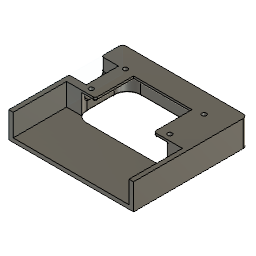
co2_fascia (Autodesk Fusion 360 design; units mm, degrees)
part number: 2026-03-11-11-56-11-354
Autodesk Fusion 360 part; units mm, degrees
note: some values were not read from the file. Chosen so that the rebuilt part matches the saved one: which face or edge a step refers to. Set by a fixed rule: which sketch regions a step uses.
sketch "Sketch1" plane through (0, 0, 0) normal (0, 0, 1) x (1, 0, 0)
  line L0 (0, 0) -> (62, 0)
  line L1 (62, 0) -> (62, 56.5)
  line L2 (62, 56.5) -> (0, 56.5)
  line L3 (0, 56.5) -> (0, 0)
  dimension "d1" = 62
  dimension "d2" = 56.5
  constraint horizontal L0
  constraint vertical L1
  constraint horizontal L2
  constraint vertical L3
  constraint coincident L0.start L3.end
  measures "d1" distance of L0.start L0.end
  measures "d2" distance of L0.start L2.end
extrude "Extrude1" add sketch "Sketch1" along normal blind 13
sketch "Sketch2" plane through (0, 0, 13) normal (0, 0, 1) x (-1, 0, 0)
  line L0 (0, -56.5) -> (0, 0)
  line L1 (0, 0) -> (-62, 0)
  line L2 (-62, 0) -> (-62, -56.5)
  line L3 (-62, -56.5) -> (0, -56.5)
  line L4 (-2.25, -26.5) -> (-59.75, -26.5)
  line L5 (-59.75, -26.5) -> (-59.75, 0.5)
  line L6 (-59.75, 0.5) -> (-2.25, 0.5)
  line L7 (-2.25, 0.5) -> (-2.25, -26.5)
  dimension "d5" = 57.5
  dimension "d6" = 27
  dimension "d7" = 30
  dimension "d8" = 2.25
  constraint horizontal L4
  constraint vertical L5
  constraint horizontal L6
  constraint vertical L7
  measures "d5" distance of L4.start L4.end
  measures "d6" distance of L4.start L6.end
  measures "d7" distance of L3 L4
  measures "d8" distance of L0 L7
extrude "Extrude2" cut sketch "Sketch2" against normal blind 11 contours L1 L4 L5 L7 | L1 L5 L6 L7
sketch "Sketch3" plane through (0, 0, 13) normal (0, 0, 1) x (-1, 0, 0)
  line L0 (-59.75, -26.5) -> (-59.75, 0)
  line L1 (-59.75, 0) -> (-62, 0)
  line L2 (-62, 0) -> (-62, -56.5)
  line L3 (-62, -56.5) -> (0, -56.5)
  line L4 (0, -56.5) -> (0, 0)
  line L5 (0, 0) -> (-2.25, 0)
  line L6 (-2.25, 0) -> (-2.25, -26.5)
  line L7 (-2.25, -26.5) -> (-59.75, -26.5)
  point P0 (-11.5, -46.5)
  point P1 (-50.5, -46.5)
  point P2 (-11.5, -29.5)
  point P3 (-50.5, -29.5)
  dimension "d11" = 10
  dimension "d12" = 11.5
  dimension "d15" = -39
  dimension "d16" = 17
  measures "d11" distance of L3 P0
  measures "d12" distance of L4 P0
hole "Hole1" at (50.5, 46.5, 13) at (50.5, 29.5, 13) at (11.5, 29.5, 13) at (11.5, 46.5, 13) direction (0, 0, -1) diameter 2.2 end through all
sketch "Sketch4" plane through (0, 0, 0) normal (0, 0, -1) x (1, 0, 0)
  circle A0 centre (11.5, -29.5) radius 1.1
  circle A1 centre (50.5, -46.5) radius 1.1
  circle A2 centre (50.5, -29.5) radius 1.1
  circle A3 centre (11.5, -46.5) radius 1.1
  line L0 (0, 0) -> (0, -56.5)
  line L1 (0, -56.5) -> (62, -56.5)
  line L2 (62, -56.5) -> (62, 0)
  line L3 (62, 0) -> (0, 0)
  line L4 (47.75, -51.275) -> (14.2, -51.275)
  line L5 (7.7, -44.775) -> (7.7, -31.225)
  line L6 (14.2, -24.725) -> (47.75, -24.725)
  line L7 (54.25, -31.225) -> (54.25, -44.775)
  arc A4 (47.75, -51.275) -> (54.25, -44.775) centre (47.75, -44.775) ccw
  arc A5 (7.7, -44.775) -> (14.2, -51.275) centre (14.2, -44.775) ccw
  arc A6 (14.2, -24.725) -> (7.7, -31.225) centre (14.2, -31.225) ccw
  arc A7 (54.25, -31.225) -> (47.75, -24.725) centre (47.75, -31.225) ccw
  point P0 (54.25, -51.275)
  point P1 (7.7, -51.275)
  point P2 (54.25, -24.725)
  dimension "d19" = 46.55
  dimension "d20" = 26.55
  dimension "d21" = 7.75
  dimension "d22" = 4.775
  dimension "d35" = 6.5
  constraint horizontal L4
  constraint vertical L5
  constraint horizontal L6
  constraint vertical L7
  constraint coincident P0 L7
  constraint coincident P0 L4
  constraint tangent L7 A4
  constraint tangent L4 A4
  constraint coincident P1 L4
  constraint coincident P1 L5
  constraint tangent L4 A5
  constraint tangent L5 A5
  constraint equal A4 A5
  constraint tangent L5 A6
  constraint tangent L6 A6
  constraint equal A4 A6
  constraint coincident P2 L6
  constraint coincident P2 L7
  constraint tangent L6 A7
  constraint tangent L7 A7
  constraint equal A4 A7
  measures "d19" distance of P0 P1
  measures "d20" distance of P0 P2
  measures "d21" distance of L2 L7
  measures "d22" distance of A1.centre L4
  measures "d35" radius of A4
extrude "Extrude3" cut sketch "Sketch4" against normal blind 11 contours L4 L5 L6 L7 A4 A5 A6 A7
sketch "Sketch5" plane through (0, 0, 0) normal (-1, 0, 0) x (0, -1, 0)
  line L0 (-56.5, 0) -> (0, 0)
  line L1 (0, 0) -> (0, 13)
  line L2 (0, 13) -> (-56.5, 13)
  line L3 (-56.5, 13) -> (-56.5, 0)
sketch "Sketch7" plane through (0, 0, 0) normal (-1, 0, 0) x (0, -1, 0)
  line L0 (-30, 13) -> (-46, 13)
  line L1 (-46, 13) -> (-46, 7)
  line L2 (-44, 5) -> (-32, 5)
  line L3 (-30, 7) -> (-30, 13)
  line L4 (-56.5, 13) -> (-56.5, 0)
  arc A0 (-32, 5) -> (-30, 7) centre (-32, 7) ccw
  arc A1 (-46, 7) -> (-44, 5) centre (-44, 7) ccw
  point P0 (-30, 5)
  dimension "d30" = 16
  dimension "d31" = 8
  dimension "d32" = 10.5
  dimension "d42" = 2
  constraint horizontal L0
  constraint vertical L1
  constraint horizontal L2
  constraint vertical L3
  constraint coincident P0 L3
  constraint coincident P0 L2
  constraint tangent L3 A0
  constraint tangent L2 A0
  constraint tangent L2 A1
  constraint tangent L1 A1
  constraint equal A0 A1
  measures "d30" distance of L0.start L0.end
  measures "d31" distance of L0.start P0
  measures "d32" distance of L1 L4
  measures "d42" radius of A0
extrude "Extrude5" cut sketch "Sketch7" against normal blind 8.5
sketch "Sketch8" plane through (0, 0, 13) normal (0, 0, 1) x (-1, 0, 0)
  line L0 (-8.5, -30) -> (0, -30)
  line L1 (0, -30) -> (0, 0)
  line L2 (0, 0) -> (-2.25, 0)
  line L3 (-2.25, 0) -> (-2.25, -26.5)
  line L4 (-2.25, -26.5) -> (-59.75, -26.5)
  line L5 (-59.75, -26.5) -> (-59.75, 0)
  line L6 (-59.75, 0) -> (-62, 0)
  line L7 (-62, 0) -> (-62, -56.5)
  line L8 (-62, -56.5) -> (0, -56.5)
  line L9 (0, -56.5) -> (0, -46)
  line L10 (0, -46) -> (-8.5, -46)
  line L11 (-8.5, -46) -> (-8.5, -30)
  circle A0 centre (-11.5, -29.5) radius 1.1
  circle A1 centre (-50.5, -46.5) radius 1.1
  circle A2 centre (-50.5, -29.5) radius 1.1
  circle A3 centre (-11.5, -46.5) radius 1.1
  line L12 (-16.5, -45.5) -> (-45.5, -45.5)
  line L13 (-45.5, -45.5) -> (-45.5, -25.5)
  line L14 (-45.5, -25.5) -> (-16.5, -25.5)
  line L15 (-16.5, -25.5) -> (-16.5, -45.5)
  dimension "d36" = 29
  dimension "d37" = 20
  dimension "d38" = 11
  dimension "d39" = 16.5
  constraint horizontal L12
  constraint vertical L13
  constraint horizontal L14
  constraint vertical L15
  measures "d36" distance of L12.start L12.end
  measures "d37" distance of L12.start L14.end
  measures "d38" distance of L8 L12
  measures "d39" distance of L7 L13
extrude "Extrude6" cut sketch "Sketch8" against normal blind 2.5 contours L4 L12 L13 L15 | L4 L13 L14 L15
fillet "Fillet1" radius 2 1 edges at (62, 56.5, 6.5)
fillet "Fillet2" radius 2 1 edges at (0, 56.5, 6.5)
fillet "Fillet3" radius 1 8 edges at (7.7, 38, 0) (9.6038, 26.6288, 0) (30.975, 24.725, 0) (52.3462, 26.6288, 0) (54.25, 38, 0) (52.3462, 49.3712, 0) (30.975, 51.275, 0) (9.6038, 49.3712, 0)
fillet "Fillet4" radius 1 5 edges at (0, 30, 10) (0, 30.5858, 5.5858) (0, 38, 5) (0, 45.4142, 5.5858) (0, 46, 10)
fillet "Fillet5" radius 1 1 edges at (45.5, 36, 11)
fillet "Fillet6" radius 1 2 edges at (31.5, 45.5, 11) (16.5, 36, 11)
fillet "Fillet7" radius 1 3 edges at (12.6182, 26.5, 11) (16.2071, 26.5, 11.2929) (16.5, 26.5, 12.5)
fillet "Fillet8" radius 1 3 edges at (45.5, 26.5, 12.5) (45.7929, 26.5, 11.2929) (49.3568, 26.5, 11)
